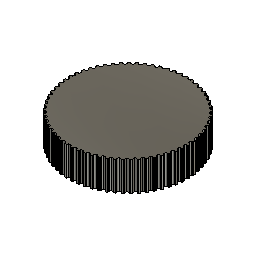
gear_65z (Autodesk Fusion 360 design; units mm, degrees)
Autodesk Fusion 360 part; units mm, degrees
sketch "Sketch1" plane through (0, 0, 0) normal (0, 0, 1) x (1, 0, 0) in component "gt2 pulley"
  circle A0 centre (0, 0) radius 20.6901 construction
  circle A1 centre (0, 0) radius 19.6861 construction
  line L0 (0, 0) -> (0, 20.6901) construction
  line L1 (0, 0) -> (0.9996, 20.666) construction
  line L2 (0, 0) -> (1.4058, 20.6423) construction
  circle A2 centre (0, 0) radius 20.4361 construction
  arc A3 (0.3927, 20.2983) -> (0.4657, 20.0037) centre (1.3886, 20.3889) ccw
  circle A4 centre (0, 0) radius 20.2861 construction
  arc A5 (0.2451, 20.4347) -> (0, 20.4361) centre (0, 0) ccw
  arc A6 (0.3927, 20.2983) -> (0.2451, 20.4347) centre (0.2433, 20.2847) ccw
  arc A7 (0.4657, 20.0037) -> (0.9511, 19.6632) centre (0.9779, 20.2175) ccw
  arc A8 (0, 20.4361) -> (-0.2451, 20.4347) centre (0, 0) ccw
  arc A9 (-0.2451, 20.4347) -> (-0.3927, 20.2983) centre (-0.2433, 20.2847) ccw
  arc A10 (-0.4657, 20.0037) -> (-0.3927, 20.2983) centre (-1.3886, 20.3889) ccw
  arc A11 (-0.9511, 19.6632) -> (-0.4657, 20.0037) centre (-0.9779, 20.2175) ccw
  arc A12 (0.9511, 19.6632) -> (-0.9511, 19.6632) centre (0, 0) ccw
  point P0 (1.3886, 20.3889)
  point P1 (0, 20.4361)
  dimension "d18" = 41.3803
  dimension "d19" = 2.769
  dimension "d22" = 1.004
  dimension "d24" = 0.75
  dimension "d26" = 1
  dimension "d27" = 0.15
  dimension "d28" = 0.15
  dimension "d47" = 0.555
  dimension "d52" = 3.812
  constraint coincident A0.centre A1.centre
  constraint coincident A0 L0.end
  constraint vertical L0
  constraint coincident A0 L1.end
  constraint coincident A0 L2.end
  constraint concentric A1 A2
  constraint coincident A1 A7.end
  constraint coincident L1 A7.end
  constraint coincident A2 P0
  constraint coincident L2 P0
  constraint coincident P0 A3.centre
  constraint coincident A2 P1
  constraint coincident L0 P1
  constraint concentric A2 A4
  constraint coincident P1 A5.end
  constraint coincident A4 A6.centre
  constraint coincident A3.start A6.start
  constraint tangent A3 A6
  constraint tangent A3 A7
  constraint symmetric L0 A7.end A11.start
  constraint symmetric L0 A3.start A9.end
  constraint symmetric L0 A3.end A10.start
  constraint symmetric L0 A3 A10
  constraint symmetric L0 A5.start A8.end
  constraint symmetric L0 P1 A5.end
  constraint symmetric L0 A5 A8
  constraint symmetric L0 A6 A9
  constraint symmetric L0 A7 A11
  constraint coincident A1 A11.start
  constraint tangent A1 A7
  constraint coincident L1 A7.centre
  measures "d18" diameter of A0
  measures "d19" angle of L0 L1
  measures "d22" distance of A0 A1
  measures "d24" distance of A1 A2
  measures "d26" radius of A3
  measures "d27" distance of A2 A4
  measures "d28" radius of A6
  measures "d47" radius of A7
extrude "Extrude1" add sketch "Sketch1" along normal blind 10 makes body 1
pattern_circular "C-Pattern1" count 65 over 360 about axis through (0, 0, 1.75) along (0, 0, 1) of bodies 1 makes body 2 at (-1.1622, 19.6518, 3.3333) makes body 3 at (-3.8859, 19.2988, 6.6667) makes body 4 at (-4.9162, 19.0624, 3.3333) makes body 5 at (-7.5213, 18.1927, 6.6667) makes body 6 at (-9.7972, 17.0751, 6.6667) makes body 7 at (-10.1618, 16.8607, 3.3333) makes body 8 at (-11.7416, 15.8012, 3.3333) makes body 9 at (-13.2118, 14.5942, 3.3333) makes body 10 at (-15.5129, 12.12, 6.6667) makes body 11 at (-15.7696, 11.784, 6.6667) makes body 12 at (-16.8333, 10.207, 3.3333) makes body 13 at (-18.0901, 7.7649, 6.6667) makes body 14 at (-18.755, 5.9827, 6.6667) makes body 15 at (-19.2449, 4.1447, 6.6667) makes body 16 at (-19.618, 1.6368, 6.6667) makes body 17 at (-19.6776, 0.5814, 6.6667) makes body 18 at (-19.6265, -1.5314, 6.6667) makes body 19 at (-19.2669, -4.0412, 6.6667) makes body 20 at (-19.1756, -4.4542, 3.3333) makes body 21 at (-18.1315, -7.6676, 6.6667) makes body 22 at (-17.3068, -9.3818, 6.6667) makes body 23 at (-16.6667, -10.4768, 6.6667) makes body 24 at (-16.0803, -11.3564, 3.3333) makes body 25 at (-14.9092, -12.8553, 3.3333) makes body 26 at (-13.5989, -14.2343, 3.3333) makes body 27 at (-11.4855, -15.9883, 6.6667) makes body 28 at (-10.6108, -16.5818, 3.3333) makes body 29 at (-8.9609, -17.5285, 3.3333) makes body 30 at (-6.4342, -18.605, 6.6667) makes body 31 at (-5.4262, -18.9235, 3.3333) makes body 32 at (-2.949, -19.464, 6.6667) makes body 33 at (-1.6894, -19.6135, 3.3333) makes body 34 at (1.0567, -19.6578, 6.6667) makes body 35 at (2.7398, -19.4946, 6.6667) makes body 36 at (4.8138, -19.0885, 6.6667) makes body 37 at (6.6336, -18.5348, 6.6667) makes body 38 at (8.3915, -17.8081, 6.6667) makes body 39 at (9.3353, -17.332, 3.3333) makes body 40 at (10.9645, -16.3501, 3.3333) makes body 41 at (12.4913, -15.2155, 3.3333) makes body 42 at (14.9092, -12.8553, 6.6667) makes body 43 at (16.0803, -11.3564, 6.6667) makes body 44 at (16.3206, -11.0084, 3.3333) makes body 45 at (17.6938, -8.6298, 6.6667) makes body 46 at (18.3691, -7.0796, 6.6667) makes body 47 at (18.7869, -5.8819, 6.6667) makes body 48 at (19.4227, -3.2101, 6.6667) makes body 49 at (19.6741, -0.6871, 6.6667) makes body 50 at (19.6827, 0.37, 6.6667) makes body 51 at (19.5296, 2.4778, 6.6667) makes body 52 at (19.1993, 4.3511, 6.6667) makes body 53 at (18.938, 5.3754, 3.3333) makes body 54 at (18.3308, 7.1781, 3.3333) makes body 55 at (17.1534, 9.6594, 6.6667) makes body 56 at (15.8953, 11.6139, 6.6667) makes body 57 at (14.978, 12.7751, 6.6667) makes body 58 at (13.6752, 14.161, 6.6667) makes body 59 at (12.8953, 14.8746, 3.3333) makes body 60 at (10.1618, 16.8607, 6.6667) makes body 61 at (9.2421, 17.3818, 6.6667) makes body 62 at (8.1035, 17.9409, 3.3333) makes body 63 at (6.3342, 18.6393, 3.3333) makes body 64 at (3.6784, 19.3394, 6.6667) makes body 65 at (2.6351, 19.509, 6.6667)
sketch "Sketch2" plane through (0, 0, 10) normal (0, 0, 1) x (-1, 0, 0)
  arc A0 (-18.7661, -7.7464) -> (-18.8322, -7.9362) centre (-18.694, -7.8779) ccw
  arc A1 (-18.8322, -7.9362) -> (-18.6365, -8.3855) centre (0, 0) ccw
  arc A2 (-18.6365, -8.3855) -> (-18.4525, -8.4664) centre (-18.4997, -8.3241) ccw
  arc A3 (-18.1533, -8.4158) -> (-18.4525, -8.4664) centre (-18.1378, -9.4157) ccw
  arc A4 (-17.6472, -8.7247) -> (-18.1533, -8.4158) centre (-18.1447, -8.9707) ccw
  arc A5 (-18.4069, -6.9808) -> (-17.6472, -8.7247) centre (0, 0) ccw
  arc A6 (-18.5253, -7.5618) -> (-18.4069, -6.9808) centre (-18.9258, -7.1776) ccw
  arc A7 (-18.7661, -7.7464) -> (-18.5253, -7.5618) centre (-19.2469, -6.8696) ccw
  circle A8 centre (0, 0) radius 19.6861
  constraint coincident A1.centre A5.centre
extrude "Extrude2" add sketch "Sketch2" against normal blind 10 contours A5 A8 bodies 1 2 3 4 5 6 7 8 9 10 11 12 13 14 15 16 17 18 19 20 21 22 23 24 25 26 27 28 29 30 31 32 33 34 35 36 37 38 39 40 41 42 43 44 45 46 47 48 49 50 51 52 53 54 55 56 57 58 59 60 61 62 63 64 65
extrude "Extrude4" [suppressed] in component "gt2 pulley"
pattern_circular "C-Pattern7" [suppressed] in component "gt2 pulley"
extrude "Extrude3" [suppressed] in component "gt2 pulley"
pattern_circular "C-Pattern6" [suppressed] in component "gt2 pulley"
extrude "Extrude2'" [suppressed] in component "gt2 pulley"
pattern_circular "C-Pattern5" [suppressed] in component "gt2 pulley"
extrude "Extrude1'" [suppressed] in component "gt2 pulley"
pattern_circular "C-Pattern4" [suppressed] in component "gt2 pulley"
pattern_circular "C-Pattern3" [suppressed] in component "gt2 pulley"
pattern_circular "C-Pattern2" [suppressed] in component "gt2 pulley"
pattern_circular "C-Pattern1'" [suppressed] in component "gt2 pulley"
copy_body "Body->Comp1" [suppressed] in component "Component"
copy_body "Body->Comp2" [suppressed] in component "Component'"
copy_body "Body->Comp3" [suppressed] in component "Component''"
copy_body "Body->Comp4" [suppressed] in component "Component'''"
copy_body "Body->Comp5" [suppressed] in component "Component''''"
copy_body "Body->Comp6" [suppressed] in component "Component'''''"
copy_body "Body->Comp7" [suppressed] in component "Component''''''"
copy_body "Body->Comp8" [suppressed] in component "Component'''''''"
copy_body "Body->Comp9" [suppressed] in component "Component''''''''"
copy_body "Body->Comp10" [suppressed] in component "Component'''''''''"
copy_body "Body->Comp11" [suppressed] in component "Component''''''''''"
copy_body "Body->Comp12" [suppressed] in component "Component'''''''''''"
copy_body "Body->Comp13" [suppressed] in component "Component''''''''''''"
copy_body "Body->Comp14" [suppressed] in component "Component'''''''''''''"
copy_body "Body->Comp15" [suppressed] in component "Component''''''''''''''"
copy_body "Body->Comp16" [suppressed] in component "Component'''''''''''''''"
copy_body "Body->Comp17" [suppressed] in component "Component''''''''''''''''"
copy_body "Body->Comp18" [suppressed] in component "Component'''''''''''''''''"
copy_body "Body->Comp19" [suppressed] in component "Component''''''''''''''''''"
copy_body "Body->Comp20" [suppressed] in component "Component'''''''''''''''''''"
component "gt2 pulley" placed x (1, 0, 0) y (0, 1, 0) z (0, 0, 1) at (0, 0, 0)
equation "NumTeeth = 65" comment "min 20"
equation "ToothPitch = 2 mm"
equation "PullyDia = NumTeeth * ToothPitch / PI"
equation "ToothAng = ( ( 360 / NumTeeth ) * 1 deg )"
equation "TransOffsetAngle = ToothAng * 0.2"
equation "Sholulder_Radius = 0.15 mm"
equation "Root_Radius = 0.555 mm"
equation "TransRadius = 1 mm"
equation "ToolHeight = 0.75 mm"
equation "PLD = 0.254 mm"
equation "d18 = PullyDia"
equation "d19 = ToothAng / 2"
equation "d22 = PLD + ToolHeight"
equation "d24 = ToolHeight"
equation "d26 = TransRadius"
equation "d27 = Sholulder_Radius"
equation "d31 = NumTeeth"
equation "d33 = NumTeeth"
equation "d35 = NumTeeth"
equation "d37 = NumTeeth"
equation "d41 = NumTeeth"
equation "d45 = NumTeeth"
equation "d47 = Root_Radius"
equation "d50 = NumTeeth"
